fandipole (Autodesk Fusion 360 design; units mm, degrees)
Autodesk Fusion 360 part; units mm, degrees
sketch "Sketch1" plane through (0, 0, 0) normal (0, 0, 1) x (1, 0, 0)
  line L0 (2.6, -2.6) -> (28.2843, -28.2843)
  line L1 (0, 0) -> (40, 0) construction
  line L2 (0, 0) -> (0, -50)
  line L3 (-2.6, -2.6) -> (-28.2843, -28.2843)
  circle A0 centre (-0.044, 4.9998) radius 5
  line L4 (28.2843, -28.2843) -> (42.4264, -14.1421)
  line L5 (28.2843, -28.2843) -> (14.1421, -42.4264)
  line L6 (-28.2843, -28.2843) -> (-14.1421, -42.4264)
  line L7 (-28.2843, -28.2843) -> (-42.4264, -14.1421)
  line L8 (-0.044, 4.9998) -> (7.456, 4.9998)
  line L9 (7.456, 4.9998) -> (42.4264, -14.1421)
  line L10 (-7.456, 4.9998) -> (-42.4264, -14.1421)
  line L11 (6.2276, -29.8757) -> (14.1421, -42.4264)
  line L12 (-6.2276, -29.8757) -> (-14.1421, -42.4264)
  line L13 (-6.2276, -29.8757) -> (6.2276, -29.8757)
  arc A1 (7.456, 4.9998) -> (-7.5439, 4.9517) centre (-0.044, 4.9998) ccw
  circle A2 centre (3.9, -28.0757) radius 1.3
  circle A3 centre (-3.9, -28.0757) radius 1.3
  line L14 (0, -9.8757) -> (12.9142, -9.8757)
  circle A4 centre (3.9, -9.8757) radius 1.3
  circle A5 centre (-3.9, -9.8757) radius 1.3
  line L15 (0, -5.1134) -> (38.8909, -17.6777)
  line L16 (0, -5.1134) -> (17.6777, -38.8909)
  circle A6 centre (28.8909, -14.447) radius 0.7
  circle A7 centre (13.8909, -9.6011) radius 0.7
  circle A8 centre (13.0407, -30.0309) radius 0.7
  circle A9 centre (6.0854, -16.741) radius 0.7
  circle A10 centre (-13.8909, -9.6011) radius 0.7
  circle A11 centre (-28.8909, -14.447) radius 0.7
  circle A12 centre (-6.0854, -16.741) radius 0.7
  circle A13 centre (-13.0407, -30.0309) radius 0.7
  line L17 (-2.6, -29.8757) -> (-2.6, -2.6)
  line L18 (-2.6, 0.7025) -> (-2.6, 0.7561)
  line L19 (2.6, -29.8757) -> (2.6, -2.6)
  line L20 (2.6, 0) -> (2.6, 0.7561)
  point P0 (0, -20)
  dimension "d1" = 45
  dimension "d2" = 40
  dimension "d3" = 10
  dimension "d4" = 15
  dimension "d5" = 20
  dimension "d6" = 20
  dimension "d7" = 20
  dimension "d8" = 2.6
  dimension "d9" = 2.6
  dimension "d10" = 1.8
  dimension "d11" = 20
  dimension "d12" = 2.6
  dimension "d13" = 5
  dimension "d14" = 5
  dimension "d15" = 1.4
  dimension "d16" = 1.4
  dimension "d17" = 1.4
  dimension "d18" = 1.4
  dimension "d19" = 10
  dimension "d20" = 10
  dimension "d21" = 15
  dimension "d22" = 15
  constraint horizontal L1
  constraint coincident L1.start L2.start
  constraint perpendicular L1 L2
  constraint symmetric L0.end L2 L3.end
  constraint concentric A0 A1
  constraint perpendicular L0 L4
  constraint perpendicular L0 L5
  constraint symmetric L2 L4.end L7.end
  constraint symmetric L2 L5.end L6.end
  constraint coincident A0.centre L8.start
  constraint horizontal L8
  constraint symmetric L2 L8.end L10.start
  constraint coincident L2 P0
  constraint perpendicular L2 L13
  constraint coincident L10 A1.end
  constraint coincident L13 L19.start
  constraint coincident A0 L20.end
  constraint perpendicular L1 L19
  constraint symmetric L2 L19.start L17.start
  constraint symmetric L2 L20.end L18.end
  constraint symmetric L2 A2 A3
  constraint coincident L2 L14.start
  constraint perpendicular L2 L14
  constraint symmetric L2 A4 A5
  constraint coincident L2 L15.start
  constraint coincident L4 L15.end
  constraint coincident L5 L16.end
  constraint coincident L15 A6.centre
  constraint coincident L15 A7.centre
  constraint coincident L16 A8.centre
  constraint coincident L16 A9.centre
  constraint symmetric L2 A6 A11
  constraint symmetric L2 A7 A10
  constraint symmetric L2 A8 A13
  constraint symmetric L2 A9 A12
  constraint coincident A0 L18.start
  constraint collinear L17 L18
  constraint coincident L1 L20.start
  constraint collinear L19 L20
  measures "d1" angle of L0 L1
  measures "d2" distance of L1.start L0.end
  measures "d3" diameter of A0
  measures "d4" diameter of A1
  measures "d5" distance of L0.end L4.end
  measures "d6" distance of L0.end L5.end
  measures "d7" distance of L1.start P0
  measures "d8" distance of L2 L19
  measures "d9" diameter of A2
  measures "d10" distance of L13 A2.centre
  measures "d11" distance of L13 L14
  measures "d12" diameter of A4
  measures "d13" distance of L4.end L15.end
  measures "d14" distance of L5.end L16.end
  measures "d15" diameter of A6
  measures "d16" diameter of A7
  measures "d17" diameter of A8
  measures "d18" diameter of A9
  measures "d19" distance of L16.end A8.centre
  measures "d20" horizontal distance of L15.end A6.centre
  measures "d21" horizontal distance of A6.centre A7.centre
  measures "d22" distance of A8.centre A9.centre
extrude "Extrude1" add sketch "Sketch1" along normal blind 2.2 contours L0 L2 A0 L4 L8 L9 L15 A6 A7 L19 | L0 L15 L19 | L0 L4 L15 A6 A7 | L0 L14 A4 L15 L19 | L14 L15 L16 L19 | L0 L5 L14 A4 L16 A8 A9 | L2 L3 A0 L7 L8 L10 L13 A1 L17 | L2 L14 L16 | L2 L13 L14 L16 L19 | L5 L11 L13 A4 L16 A8 A9 L19 | L3 L6 L12 L13 L17
fillet "Fillet1" radius 2.5 8 edges at (42.4264, -14.1421, 1.1) (14.1421, -42.4264, 1.1) (6.2276, -29.8757, 1.1) (-6.2276, -29.8757, 1.1) (-14.1421, -42.4264, 1.1) (-42.4264, -14.1421, 1.1) (-7.5439, 4.9517, 1.1) (7.456, 4.9998, 1.1)
fillet "Fillet2" radius 1 2 edges at (-4.7056, 6.8079, 2.2) (-4.7056, 6.8079, 0)
fillet "Fillet3" radius 0.5 8 edges at (-5.112, -9.4056, 2.2) (5.1938, -9.7485, 2.2) (-5.112, -9.4056, 0) (5.1938, -9.7485, 0) (-5.112, -27.6056, 2.2) (-5.112, -27.6056, 0) (2.688, -27.6056, 2.2) (2.688, -27.6056, 0)
fillet "Fillet4" radius 0.5 16 edges at (-29.5435, -14.1939, 2.2) (-29.5435, -14.1939, 0) (-14.5435, -9.3479, 2.2) (-14.5435, -9.3479, 0) (-6.738, -16.4878, 2.2) (-6.738, -16.4878, 0) (-13.6934, -29.7778, 2.2) (-13.6934, -29.7778, 0) (5.4327, -16.4878, 2.2) (5.4327, -16.4878, 0) (12.3881, -29.7778, 2.2) (12.3881, -29.7778, 0) (13.2382, -9.3479, 2.2) (13.2382, -9.3479, 0) (28.2382, -14.1939, 2.2) (28.2382, -14.1939, 0)
